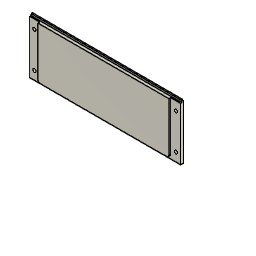
Under Table Mainboard Case - Back (Autodesk Fusion 360 design; units mm, degrees)
Autodesk Fusion 360 part; units mm, degrees
sketch "Sketch2" plane through (0, 67, 0) normal (0, 1, 0) x (-1, 0, 0)
  circle A0 centre (-79.5, 13) radius 1.425
  circle A1 centre (79.5, 53) radius 1.425
  circle A2 centre (-79.5, 53) radius 1.425
  circle A3 centre (79.5, 13) radius 1.425
  line L0 (-85, 3) -> (85, 3)
  line L1 (85, 3) -> (85, 63)
  line L2 (85, 63) -> (74, 63)
  line L3 (74, 63) -> (74, 5)
  line L4 (74, 5) -> (-74, 5)
  line L5 (-74, 5) -> (-74, 63)
  line L6 (-74, 63) -> (-85, 63)
  line L7 (-85, 63) -> (-85, 3)
  line L8 (-74, 63) -> (-71.1802, 63)
  line L9 (-84.75, 63) -> (-84.75, 3.25)
  line L10 (-84.75, 3.25) -> (84.75, 3.25)
  line L11 (84.75, 3.25) -> (84.75, 63)
  line L12 (-84.75, 63) -> (84.75, 63)
  dimension "d90" = -0.25
  constraint coincident L5.end L6.start
  constraint perpendicular L5 L8
  constraint perpendicular L11 L12
extrude "Extrude1" add sketch "Sketch2" along normal blind 3 contours L2 L3 L4 L5 L6 L9 L10 L11 L12 | L3 L4 L5 L8 L12
sketch "Sketch3" plane through (0, 67, 0) normal (0, -1, 0) x (1, 0, 0)
  circle A0 centre (79.5, 53) radius 1.425
  circle A1 centre (-79.5, 13) radius 1.425
  circle A2 centre (79.5, 13) radius 1.425
  circle A3 centre (-79.5, 53) radius 1.425
  line L0 (-84.75, 3.25) -> (84.75, 3.25)
  line L1 (84.75, 3.25) -> (84.75, 63)
  line L2 (84.75, 63) -> (-84.75, 63)
  line L3 (-84.75, 63) -> (-84.75, 3.25)
  line L4 (-74, 5) -> (-74, 63)
  line L5 (-74, 5) -> (74, 5)
  line L6 (74, 5) -> (74, 63)
  line L7 (-73.7, 5.3) -> (-73.7, 63)
  line L8 (-73.7, 5.3) -> (73.7, 5.3)
  line L9 (73.7, 5.3) -> (73.7, 63)
  dimension "d93" = -0.3
extrude "Extrude2" add sketch "Sketch3" along normal blind 2 contours L2 L7 L8 L9
fillet "Fillet1" radius 3 2 edges at (-73.7, 66, 5.3) (73.7, 66, 5.3)
sketch "Sketch4" plane through (0, 0, 63) normal (0, 0, 1) x (-1, 0, 0)
  line L0 (-73.7, -67) -> (-84.75, -67)
  line L1 (-84.75, -67) -> (-84.75, -70)
  line L2 (-84.75, -70) -> (84.75, -70)
  line L3 (84.75, -70) -> (84.75, -67)
  line L4 (84.75, -67) -> (73.7, -67)
  line L5 (73.7, -67) -> (73.7, -65)
  line L6 (73.7, -65) -> (-73.7, -65)
  line L7 (-73.7, -65) -> (-73.7, -67)
  line L8 (84.75, -68.4) -> (-84.75, -68.4)
  dimension "d97" = 1.6
  constraint coincident L3 L8.start
  constraint coincident L1 L8.end
  constraint perpendicular L1 L8
  measures "d97" distance of L2 L8
extrude "Extrude3" add sketch "Sketch4" along normal blind 2 contours L1 L2 L3 L8
sketch "Sketch5" plane through (-0.703, 70, -0.4927) normal (0, 1, 0) x (-1, 0, 0)
  circle A0 centre (-80.203, 53.4927) radius 1.425
  circle A1 centre (78.797, 13.4927) radius 1.425
  circle A2 centre (-80.203, 13.4927) radius 1.425
  circle A3 centre (78.797, 53.4927) radius 1.425
  line L0 (-85.453, 3.7427) -> (84.047, 3.7427)
  line L1 (84.047, 3.7427) -> (84.047, 65.4927)
  line L2 (84.047, 65.4927) -> (-85.453, 65.4927)
  line L3 (-85.453, 65.4927) -> (-85.453, 3.7427)
  circle A4 centre (-80.203, 53.4927) radius 1.75
  circle A5 centre (-80.203, 13.4927) radius 1.75
  circle A6 centre (78.797, 53.4927) radius 1.75
  circle A7 centre (78.797, 13.4927) radius 1.75
  dimension "d100" = 3.5
  dimension "d101" = 3.5
  dimension "d102" = 3.5
  dimension "d103" = 3.5
  constraint concentric A0 A4
  constraint concentric A2 A5
  constraint concentric A3 A6
  constraint concentric A1 A7
  measures "d100" diameter of A4
  measures "d101" diameter of A5
  measures "d102" diameter of A6
  measures "d103" diameter of A7
extrude "Extrude4" cut sketch "Sketch5" against normal blind 3 contours A4 | A5 | A6 | A7
